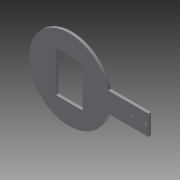
# Autodesk Inventor part: 零件2
Saved by Autodesk Inventor 2014 (Build 180170000, 170)
## iProperties
Created: 2024-03-26
Part Number: 零件2
Material: 常规
Document SubType Name: Modeling
Designer: Administrator
Density: 1 g/cm^3
Appearance: 默认
Author: Administrator
Autodesk Inventor part; units mm, degrees
ref_plane "YZ Plane" through (0, 0, 0) normal (1, 0, 0) x (0, 1, 0)
ref_plane "XZ Plane" through (0, 0, 0) normal (0, 1, 0) x (-1, 0, 0)
ref_plane "XY Plane" through (0, 0, 0) normal (0, 0, 1) x (1, 0, 0)
sketch "草图1" plane through (0, 0, 0) normal (0, 1, 0) x (-1, 0, 0)
  arc A0 (-58.0948, -15) -> (-58.0948, 15) centre (0, 0) ccw
  line L0 (0, -30) -> (20, -30)
  line L1 (20, -30) -> (20, 30)
  line L2 (20, 30) -> (-20, 30)
  line L3 (-20, 30) -> (-20, -30)
  line L4 (-20, -30) -> (0, -30)
  line L5 (-58.0948, -15) -> (-118.0948, -15)
  line L6 (-118.0948, -15) -> (-118.0948, 15)
  line L7 (-118.0948, 15) -> (-58.0948, 15)
  circle A1 centre (-94.0948, 0) radius 1.5
  circle A2 centre (-114.0948, 0) radius 1.5
  dimension "d12" = 30
  dimension "d15" = 3
  dimension "d16" = 3
  constraints: 16 end point, 3 centre point, 2 parallel, 2 point on circle, 1 coincident, 1 collinear, 1 perpendicular
  measures "d12" distance of L5.end L6.end
  measures "d15" diameter of A1
  measures "d16" diameter of A2
extrude "拉伸1" add sketch "草图1" along normal blind 4
